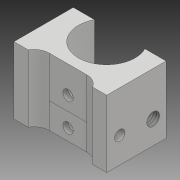
# Autodesk Inventor part: trolley
Saved by Autodesk Inventor 2017 SP1 (Build 210196100, 196)
## iProperties
Created: 2018-01-19
Part Number: trolley
Material: Generic
Document SubType Name: Modeling
Designer: Tomasz
Density: 1 g/cm^3
Appearance: Default
Author: Tomasz
Autodesk Inventor part; units mm, degrees
ref_plane "YZ Plane" through (0, 0, 0) normal (1, 0, 0) x (0, 1, 0)
ref_plane "XZ Plane" through (0, 0, 0) normal (0, 1, 0) x (-1, 0, 0)
sketch "Sketch1" plane through (0, 0, 0) normal (0, 0, 1) x (1, 0, 0)
  arc A0 (-4.3301, 2.5) -> (4.3301, 2.5) centre (0, 0) ccw
  line L0 (-4.3301, 2.5) -> (-9, 2.5)
  line L1 (-9, 2.5) -> (-9, -9)
  line L2 (-9, -9) -> (-6.25, -9)
  line L3 (-3.6519, -7.5) -> (3.6519, -7.5)
  line L4 (6.25, -9) -> (9, -9)
  line L5 (9, -9) -> (9, 2.5)
  line L6 (9, 2.5) -> (4.3301, 2.5)
  line L7 (0, 15.116) -> (0, -11.4442) construction
  arc A1 (-3.6519, -7.5) -> (-6.25, -9) centre (-3.6519, -10.5) ccw
  arc A2 (6.25, -9) -> (3.6519, -7.5) centre (3.6519, -10.5) ccw
  dimension "d0" = 10
  dimension "d2" = 7.5
  dimension "d5" = 18
  dimension "d6" = 2.5
  dimension "d7" = 6
  dimension "d8" = 6
  dimension "d9" = 12.5
  dimension "d10" = 1.5
  constraints: 16 end point, 6 point on circle, 5 point on line, 3 centre point, 2 horizontal, 2 perpendicular, 1 coincident, 1 symmetric about line, 1 tangent, 1 vertical, 1 other
  measures "d0" diameter of A0
  measures "d2" distance from line of L3 point (0, 0)
  measures "d5" distance between parallel lines of L5 L1
  measures "d6" distance from line of point (0, 0) L0
  measures "d7" diameter of A1
  measures "d8" diameter of A2
  measures "d9" distance of L4.start L2.end
  measures "d10" distance between parallel lines of L2 L3
sketch "Sketch2" plane through (0, 0, 0) normal (0, 0, 1) x (1, 0, 0)
  line L0 (-4.3301, 2.5) -> (-9, 2.5) projected
  line L1 (-9, 2.5) -> (-9, -9) projected
  line L2 (-9, -9) -> (-6.25, -9) projected
  arc A0 (-3.6519, -7.5) -> (-6.25, -9) centre (-3.6519, -10.5) ccw projected
  line L3 (-3.6519, -7.5) -> (3.6519, -7.5) projected
  arc A1 (6.25, -9) -> (3.6519, -7.5) centre (3.6519, -10.5) ccw projected
  line L4 (6.25, -9) -> (9, -9) projected
  line L5 (9, -9) -> (9, 2.5) projected
  line L6 (9, 2.5) -> (4.3301, 2.5) projected
  arc A2 (-4.3301, 2.5) -> (4.3301, 2.5) centre (0, 0) ccw projected
extrude "Extrusion1" add sketch "Sketch2" along normal blind 13
sketch "Sketch3" plane through (0, 0, 13) normal (0, 0, 1) x (1, 0, 0)
  circle A0 centre (0, 0) radius 5.5
  dimension "d13" = 11
  constraints: 1 centre point, 1 coincident
  measures "d13" diameter of A0
extrude "Extrusion2" cut sketch "Sketch3" against normal blind 12
sketch "Sketch4" plane through (-9, 2.5, 0) normal (0, 1, 0) x (1, 0, 0)
  line L0 (9, 0) -> (9, -15.5) construction
  line L1 (18, -13) -> (13.899, -13) projected
  line L2 (14.5, -13) -> (3.5, -13) projected
  point P0 (9, -2.25)
  point P1 (9, -7.75)
  point P2 (16.25, -8.25)
  point P3 (4.101, -13)
  dimension "d16" = 7.25
  dimension "d17" = 4.75
  dimension "d18" = 5.25
  dimension "d19" = 5.5
  constraints: 2 end point, 1 midpoint, 1 point on line, 1 vertical
  measures "d16" distance from line of point (16.25, -8.25) L0
  measures "d17" distance from line of L1 point (16.25, -8.25)
  measures "d18" distance from line of point (9, -7.75) L2
  measures "d19" distance of point (9, -7.75) point (9, -2.25)
sketch "Sketch5" plane through (4.3301, 2.5, 0) normal (0, 1, 0) x (1, 0, 0)
  point P0 (-4.3301, 0)
  point P1 (2.9199, -8.25)
hole "Hole1" at (7.25, 2.5, 8.25) direction (0, -1, 0) diameter 1.5 depth 5 tip angle 118
ref_plane "Work Plane1" through (0, -5.5, 13) normal (0, 1, 0) x (-1, 0, 0)
sketch "Sketch6" plane through (-9, 2.5, 0) normal (0, 1, 0) x (1, 0, 0)
  point P0 (9, 0)
  point P1 (9, -2.25)
  point P2 (9, -7.75)
hole "Hole2" at (0, 2.5, 7.75) at (0, 2.5, 2.25) direction (0, -1, 0) diameter 4 depth 8
sketch "Sketch7" plane through (0, -5.5, 13) normal (0, 1, 0) x (-1, 0, 0)
  point P0 (0, -13)
  point P1 (0, -10.75)
  point P2 (0, -5.25)
hole "Hole3" at (0, -5.5, 2.25) at (0, -5.5, 7.75) direction (0, -1, 0) diameter 2 end through all countersink diameter 4 countersink angle 90
sketch "Sketch8" plane through (-9, -9, 0) normal (-1, 0, 0) x (0, 0, 1)
  line L0 (0, 11.5) -> (13, 11.5) projected
  line L1 (0, 11.5) -> (0, 0) projected
  point P0 (0, 9)
  point P1 (5, 2.5)
  point P2 (4.5, 9)
  dimension "d41" = 9
  dimension "d42" = 5
  dimension "d43" = 2.5
  dimension "d44" = 4.5
  measures "d41" distance from line of point (5, 2.5) L0
  measures "d42" distance from line of point (5, 2.5) L1
  measures "d43" distance from line of point (4.5, 9) L0
  measures "d44" distance from line of point (4.5, 9) L1
sketch "Sketch9" plane through (-9, -9, 0) normal (-1, 0, 0) x (0, 0, 1)
  point P0 (0, 9)
  point P1 (5, 2.5)
hole "Hole4" at (-9, -6.5, 5) direction (1, 0, 0) diameter 2 end through all
sketch "Sketch10" plane through (-9, -9, 0) normal (-1, 0, 0) x (0, 0, 1)
  point P0 (0, 9)
  point P1 (4.5, 9)
hole "Hole5" at (-9, 0, 4.5) direction (1, 0, 0) diameter 2.459 end through all thread size "M3x0.5" class "6H" standard "ANSI Metric M Profile"
equation "\"d7\" = d8"
body "Solid1"
